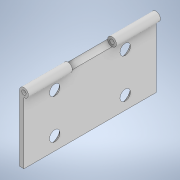
# Autodesk Inventor part: hinge 2
Saved by Autodesk Inventor 2021 (Build 250183000, 183)
## iProperties
Created: 2021-01-11
Part Number: hinge 2
Material: Ogólny
Document SubType Name: Modeling
Designer: Adam
Density: 1 g/cm^3
Appearance: Domyślna
Author: Adam
Autodesk Inventor part; units mm, degrees
ref_plane "YZ Plane" through (0, 0, 0) normal (1, 0, 0) x (0, 1, 0)
ref_plane "XZ Plane" through (0, 0, 0) normal (0, 1, 0) x (-1, 0, 0)
ref_plane "XY Plane" through (0, 0, 0) normal (0, 0, 1) x (1, 0, 0)
sketch "Szkic1" plane through (0, 0, 0) normal (0, 0, 1) x (1, 0, 0)
  line L0 (2, 10) -> (1, 10)
  line L1 (1, 10) -> (1, -5)
  line L2 (1, -5) -> (2, -5)
  line L3 (2, -5) -> (2, 10)
  circle A0 centre (2, 10) radius 1
  point P0 (0, 0)
  point P1 (0, 0)
  point P2 (2, 9)
  point P3 (2, 9)
  constraints: 8 end point, 2 parallel, 1 centre point, 1 coincident, 1 horizontal, 1 perpendicular, 1 tangent
extrude "Wyciągnięcie proste1" add sketch "Szkic1" along normal blind 30
ref_plane "Płaszczyzna konstrukcyjna1" through (0, 0, 10) normal (0, 0, 1) x (1, 0, 0)
sketch "Szkic2" plane through (0, 0, 10) normal (0, 0, 1) x (1, 0, 0)
  arc A0 (2, 9) -> (1, 10) centre (2, 10) ccw projected
  circle A1 centre (2, 10) radius 1
  point P0 (0, 0)
  constraints: 3 other
extrude "Wyciągnięcie proste2" cut sketch "Szkic2" along normal blind 10
sketch "Szkic3" plane through (0, 0, 30) normal (0, 0, 1) x (1, 0, 0)
  circle A0 centre (2, 10) radius 0.5
  point P0 (0, 0)
  dimension "d5" = 1
  constraints: 1 centre point
  measures "d5" diameter of A0
extrude "Wyciągnięcie proste3" cut sketch "Szkic3" against normal blind 30
sketch "Szkic8" plane through (1, -5, 0) normal (-1, 0, 0) x (0, 0, 1)
  point P0 (7, 3)
hole "Otwór5" at (1, -2, 7) direction (1, 0, 0) diameter 2.4 end through all countersink diameter 4.4 countersink angle 90
sketch "Szkic9" plane through (1, -5, 0) normal (-1, 0, 0) x (0, 0, 1)
  point P0 (7, 12)
hole "Otwór6" at (1, 7, 7) direction (1, 0, 0) diameter 2.4 end through all countersink diameter 4.4 countersink angle 90
sketch "Szkic10" plane through (1, -5, 0) normal (-1, 0, 0) x (0, 0, 1)
  point P0 (23, 12)
hole "Otwór7" at (1, 7, 23) direction (1, 0, 0) diameter 2.4 end through all countersink diameter 4.4 countersink angle 90
sketch "Szkic11" plane through (1, -5, 0) normal (-1, 0, 0) x (0, 0, 1)
  point P0 (23, 3)
hole "Otwór8" at (1, -2, 23) direction (1, 0, 0) diameter 2.4 end through all countersink diameter 4.4 countersink angle 90
